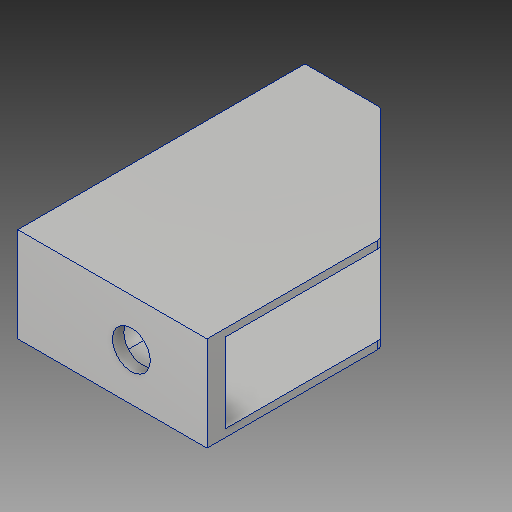
# Autodesk Inventor part: Top Connector
Saved by Autodesk Inventor 2019.4 (Build 234330000, 330)
## iProperties
Created: 2020-01-09
Part Number: Top Connector
Material: Aluminum 6061
Document SubType Name: Modeling
Designer: Mark
Density: 2.7 g/cm^3
Appearance: Aluminum - Flat
Mass: 109.502 g
Surface Area: 167.933 cm^2
Volume: 40.5563 cm^3
Author: Mark
Autodesk Inventor part; units mm, degrees
ref_plane "YZ Plane" through (0, 0, 0) normal (1, 0, 0) x (0, 1, 0)
ref_plane "XZ Plane" through (0, 0, 0) normal (0, 1, 0) x (-1, 0, 0)
ref_plane "XY Plane" through (0, 0, 0) normal (0, 0, 1) x (1, 0, 0)
sketch "Sketch1" plane through (0, 0, 0) normal (0, 0, 1) x (1, 0, 0)
  circle A0 centre (0, 0) radius 10.15
  line L0 (-20, -12.5) -> (20, -12.5)
  line L1 (20, -12.5) -> (20, 12.5)
  line L2 (20, 12.5) -> (-20, 12.5)
  line L3 (-20, 12.5) -> (-20, -12.5)
  line L4 (-20, -12.5) -> (20, 12.5) construction
  line L5 (20, -12.5) -> (-20, 12.5) construction
  dimension "d0" = 20.3
  dimension "d1" = 40
  dimension "d2" = 25
  constraints: 12 end point, 2 midpoint, 2 parallel, 1 centre point, 1 coincident, 1 horizontal, 1 perpendicular
  measures "d0" diameter of A0
  measures "d1" distance of L2.end L1.end
  measures "d2" distance of L1.end L0.end
extrude "Extrusion1" add sketch "Sketch1" along normal blind 2
sketch "Sketch2" plane through (0, 0, 2) normal (0, 0, 1) x (1, 0, 0)
  circle A0 centre (0, 0) radius 5
  line L0 (20, -12.5) -> (20, 12.5) projected
  line L1 (-20, -12.5) -> (20, -12.5)
  line L2 (20, -12.5) -> (20, 12.5)
  line L3 (20, 12.5) -> (-20, 12.5)
  line L4 (-20, 12.5) -> (-20, -12.5)
  line L5 (-20, -12.5) -> (20, 12.5) construction
  line L6 (20, -12.5) -> (-20, 12.5) construction
  dimension "d5" = 10
  dimension "d6" = 40
  dimension "d7" = 25
  constraints: 12 end point, 2 midpoint, 2 parallel, 1 centre point, 1 coincident, 1 horizontal, 1 perpendicular
  measures "d5" diameter of A0
  measures "d6" distance of L3.end L0.end
  measures "d7" distance of L0.end L1.end
extrude "Extrusion2" add sketch "Sketch2" along normal blind 3
sketch "Sketch3" plane through (0, 0, 0) normal (0, 0, -1) x (-1, 0, 0)
  line L0 (-20, 12.5) -> (20, 12.5) projected
  line L1 (20, 12.5) -> (15, 12.5)
  line L2 (15, 12.5) -> (15, -12.5)
  line L3 (15, -12.5) -> (20, -12.5)
  line L4 (20, -12.5) -> (20, 12.5)
  line L5 (15, 12.5) -> (-20, 12.5)
  line L6 (-20, 12.5) -> (-20, 10.5)
  line L7 (-20, 10.5) -> (15, 10.5)
  line L8 (15, 10.5) -> (15, 12.5)
  line L9 (15, -12.5) -> (-20, -12.5)
  line L10 (-20, -12.5) -> (-20, -10.5)
  line L11 (-20, -10.5) -> (15, -10.5)
  line L12 (15, -10.5) -> (15, -12.5)
  point P0 (0, 0)
  dimension "d10" = 5
  dimension "d11" = 25
  dimension "d12" = 35
  dimension "d13" = 2
  dimension "d14" = 35
  dimension "d15" = 2
  constraints: 24 end point, 6 parallel, 3 horizontal, 3 perpendicular
  measures "d10" distance of L3.end L2.end
  measures "d11" distance of L2.end L1.end
  measures "d12" distance of L7.end L6.end
  measures "d13" distance of L6.end L5.end
  measures "d14" distance of L10.end L11.end
  measures "d15" distance of L9.end L10.end
extrude "Extrusion3" add sketch "Sketch3" along normal blind 70.88
chamfer "Chamfer1" distance 30 angle 45 2 edges at (20, 11.5, -70.88) (20, -11.5, -70.88)
fillet "Fillet1" radius 4 2 edges at (-15, 10.5, -35.44) (-15, -10.5, -35.44)
fillet "Fillet2" radius 2 4 edges at (-10, -11.5, -70.88) (-10, 11.5, -70.88) (20, -11.5, -40.88) (20, 11.5, -40.88)
sketch "Sketch5" plane through (-20, -12.5, 5) normal (-1, 0, 0) x (0, 0, 1)
  line L0 (0, 0) -> (-75.88, 0) projected
  line L1 (-45.0516, 25) -> (0, 25) projected
  line L2 (-75.88, 0) -> (0, 0)
  line L3 (0, 0) -> (0, 25)
  line L4 (0, 25) -> (-75.88, 25)
  line L5 (-75.88, 25) -> (-75.88, 0)
  point P0 (-5, 12.5)
  constraints: 8 end point, 2 parallel, 1 horizontal, 1 perpendicular
extrude "Extrusion5" add sketch "Sketch5" along normal blind 10
body "Solid1"
